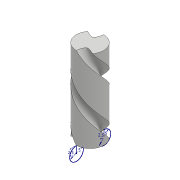
# Autodesk Inventor part: screw
Saved by Autodesk Inventor 2018 (Build 220112000, 112)
## iProperties
Created: 2018-08-17
Part Number: screw
Material: Generic
Document SubType Name: Modeling
Designer: Bardo91
Density: 1 g/cm^3
Appearance: Default
Author: Bardo91
Autodesk Inventor part; units mm, degrees
ref_plane "YZ Plane" through (0, 0, 0) normal (1, 0, 0) x (0, 1, 0)
ref_plane "XZ Plane" through (0, 0, 0) normal (0, 1, 0) x (-1, 0, 0)
ref_plane "XY Plane" through (0, 0, 0) normal (0, 0, 1) x (1, 0, 0)
sketch "Sketch1" plane through (0, 0, 0) normal (0, 0, 1) x (1, 0, 0)
  circle A0 centre (0, 0) radius 5
  dimension "d0" = 10
  constraints: 1 centre point, 1 coincident
  measures "d0" diameter of A0
extrude "Extrusion1" add sketch "Sketch1" along normal blind 30
sketch "Sketch2" plane through (0, 0, 0) normal (1, 0, 0) x (0, 1, 0)
  line L0 (-5, 0) -> (5, 0) projected
  line L1 (5, 0) -> (5, -2.5)
  circle A0 centre (5, -2.5) radius 2.5
  line L2 (-5, 0) -> (-5, -2.5)
  circle A1 centre (-5, -2.5) radius 2.5
  point P0 (0, 0)
  dimension "d3" = 2.5
  dimension "d4" = 5
  dimension "d5" = 2.5
  dimension "d6" = 5
  constraints: 4 end point, 2 centre point, 2 coincident, 2 vertical
  measures "d3" distance of L0.end L1.end
  measures "d4" diameter of A0
  measures "d5" distance of L0.start L2.end
  measures "d6" diameter of A1
coil "Coil1" sketch "Sketch2" operation cut axis through (0, 0, -10) along (0, 0, 1) pitch 35 turns 1 hand left contours A0
coil "Coil2" sketch "Sketch2" operation cut axis through (0, 0, -10) along (0, 0, 1) pitch 35 turns 1 hand left contours A1
body "Solid1"
